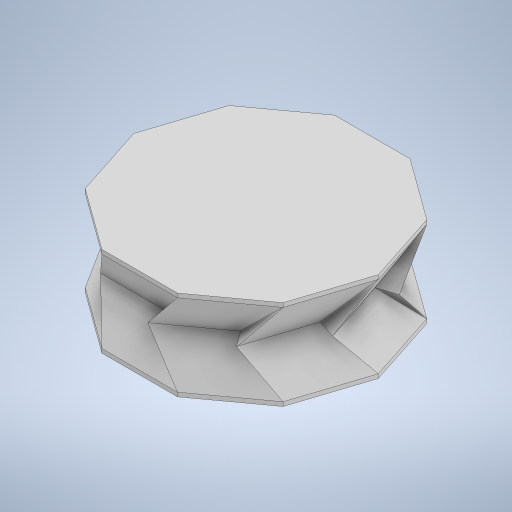
# Autodesk Inventor part: OV-PAM_n_10_standard_1F
Saved by Autodesk Inventor 2024 (Build 280153000, 153)
## iProperties
Created: 2023-08-31
Part Number: OV-PAM_n_10_standard_1F
Material: 일반
Document SubType Name: Modeling
Designer: jsw
Density: 1 g/cm^3
Appearance: 기본값
Author: jsw
Autodesk Inventor part; units mm, degrees
ref_plane "YZ Plane" through (0, 0, 0) normal (1, 0, 0) x (0, 1, 0)
ref_plane "XZ Plane" through (0, 0, 0) normal (0, 1, 0) x (-1, 0, 0)
ref_plane "XY Plane" through (0, 0, 0) normal (0, 0, 1) x (1, 0, 0)
sketch "스케치1" plane through (0, 0, 0) normal (0, 1, 0) x (-1, 0, 0)
  line L0 (-10.9012, 33.5504) -> (10.9012, 33.5504)
  line L1 (10.9012, 33.5504) -> (28.5397, 20.7353)
  line L2 (28.5397, 20.7353) -> (35.277, 0)
  line L3 (35.277, 0) -> (28.5397, -20.7353)
  line L4 (28.5397, -20.7353) -> (10.9012, -33.5504)
  line L5 (10.9012, -33.5504) -> (-10.9012, -33.5504)
  line L6 (-10.9012, -33.5504) -> (-28.5397, -20.7353)
  line L7 (-28.5397, -20.7353) -> (-35.277, 0)
  line L8 (-35.277, 0) -> (-28.5397, 20.7353)
  line L9 (-28.5397, 20.7353) -> (-10.9012, 33.5504)
  line L10 (11.0961, -34.1504) -> (-11.0961, -34.1504)
  line L11 (-11.0961, -34.1504) -> (-29.0501, -21.1061)
  line L12 (-29.0501, -21.1061) -> (-35.9079, 0)
  line L13 (-35.9079, 0) -> (-29.0501, 21.1061)
  line L14 (-29.0501, 21.1061) -> (-11.0961, 34.1504)
  line L15 (-11.0961, 34.1504) -> (11.0961, 34.1504)
  line L16 (11.0961, 34.1504) -> (29.0501, 21.1061)
  line L17 (29.0501, 21.1061) -> (35.9079, 0)
  line L18 (35.9079, 0) -> (29.0501, -21.1061)
  line L19 (29.0501, -21.1061) -> (11.0961, -34.1504)
  point P0 (0, 0)
  point P1 (0, 0)
  point P2 (0, 0)
  dimension "d0" = 70.554
  dimension "d1" = 0.6
  constraints: 40 end point, 2 coincident, 2 horizontal, 42 other
  measures "d0" distance of L0.start L4.end
  measures "d1" distance between parallel lines of L5 L10
extrude "돌출1" add sketch "스케치1" along normal blind 12 contours L0 L1 L2 L3 L4 L5 L6 L7 L8 L9 | L10 L11 L12 L13 L14 L15 L16 L17 L18 L19
ref_plane "작업 평면1" through (29.0501, 0, 21.1061) normal (-0.8236391, -0.5, -0.2676166) x (0.309017, 0, -0.9510565)
sketch "스케치2" plane through (35.9079, 0, 0) normal (0.9510565, 0, 0.309017) x (0.309017, 0, -0.9510565)
  line L0 (-22.1923, 0) -> (0, 0) projected
  line L1 (0, 0) -> (0, 12) projected
  line L2 (-22.1923, 12) -> (0, 12) projected
  line L3 (-22.1923, 0) -> (-22.1923, 12) projected
  line L4 (-22.1923, 0) -> (-40.1462, 0) projected
  line L5 (-22.1923, 0) -> (-36.4933, 12)
  line L6 (-22.1923, 12) -> (-40.1462, 12) projected
  line L7 (0, 0) -> (-10, 12)
  point P0 (-11.0961, 0)
  dimension "d5" = 140
  dimension "d6" = 10
  constraints: 4 end point, 2 point on line
  measures "d5" angle of L5 L0
  measures "d6" distance of L1.end L7.end
extrude "돌출2" cut sketch "스케치2" against normal up to surface contours L3 L2 L7 L0 | L5 L6 L3 surface through (29.0501, 0, 21.1061) normal (-0.8236391, -0.5, -0.2676166)
pattern_circular "원형 패턴1" count 10 over 360 about axis through (0, -10, 0) along (0, 1, 0) of "돌출2"
sketch "스케치3" plane through (0, 0, 0) normal (0, -1, 0) x (1, 0, 0)
  line L0 (-29.0501, -21.1061) -> (-35.9079, 0) projected
  line L1 (-11.0961, -34.1504) -> (-29.0501, -21.1061) projected
  line L2 (11.0961, -34.1504) -> (-11.0961, -34.1504) projected
  line L3 (29.0501, -21.1061) -> (11.0961, -34.1504) projected
  line L4 (35.9079, 0) -> (29.0501, -21.1061) projected
  line L5 (29.0501, 21.1061) -> (35.9079, 0) projected
  line L6 (11.0961, 34.1504) -> (29.0501, 21.1061) projected
  line L7 (-11.0961, 34.1504) -> (11.0961, 34.1504) projected
  line L8 (-29.0501, 21.1061) -> (-11.0961, 34.1504) projected
  line L9 (-35.9079, 0) -> (-29.0501, 21.1061) projected
  point P0 (0, 0)
extrude "돌출3" add sketch "스케치3" along normal blind 1.2
ref_plane "작업 평면2" through (0, 12, 0) normal (0, 1, 0) x (1, 0, 0)
mirror "미러1" about plane through (0, 12, 0) normal (0, 1, 0) of "돌출3", "돌출2", "원형 패턴1", "돌출1"
